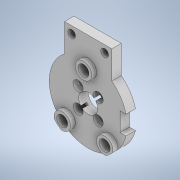
# Autodesk Inventor part: Spacerplate
Saved by Autodesk Inventor 2021 (Build 250183000, 183)
## iProperties
Created: 2024-03-24
Part Number: Spacerplate
Material: Generic
Document SubType Name: Modeling
Designer: Lukas
Density: 1 g/cm^3
Appearance: Default
Author: Lukas
Autodesk Inventor part; units mm, degrees
ref_plane "YZ Plane" through (0, 0, 0) normal (1, 0, 0) x (0, 1, 0)
ref_plane "XZ Plane" through (0, 0, 0) normal (0, 1, 0) x (-1, 0, 0)
ref_plane "XY Plane" through (0, 0, 0) normal (0, 0, 1) x (1, 0, 0)
sketch "Sketch1" plane through (0, 0, 0) normal (0, 0, 1) x (1, 0, 0)
  circle A0 centre (0, 0) radius 16.5
  circle A1 centre (-4.25, 4.25) radius 1.2
  circle A2 centre (-4.25, -4.25) radius 1.2
  circle A3 centre (4.25, -4.25) radius 1.2
  circle A4 centre (4.25, 4.25) radius 1.2
  circle A5 centre (0, 0) radius 4
  circle A6 centre (0, 13) radius 2.3
  circle A7 centre (-9, -10) radius 2.3
  circle A8 centre (9, -10) radius 2.3
  line L0 (16.5, -4) -> (13.5, -4)
  line L1 (13.5, -4) -> (13.5, 4)
  line L2 (13.5, 4) -> (16.5, 4)
  line L3 (16.5, 4) -> (16.5, -4)
  line L4 (-10, 13.1244) -> (-10, 25)
  line L5 (-10, 25) -> (10, 25)
  line L6 (10, 25) -> (10, 13.1244)
  circle A9 centre (7, 22) radius 1.6
  circle A10 centre (-7, 22) radius 1.6
  point P0 (13.5, 0)
  point P1 (16.0078, 4)
  point P2 (16.0078, -4)
  point P3 (0, 25)
  dimension "d0" = 33
  dimension "d1" = 8.5
  dimension "d2" = 8.5
  dimension "d3" = 4.25
  dimension "d4" = 4.25
  dimension "d5" = 2.4
  dimension "d6" = 8
  dimension "d7" = 13
  dimension "d8" = 4.6
  dimension "d9" = 10
  dimension "d10" = 9
  dimension "d11" = 9
  dimension "d17" = 3
  dimension "d18" = 8
  dimension "d27" = 25
  dimension "d28" = 20
  dimension "d30" = 3.2
  dimension "d31" = 14
  dimension "d32" = 7
  dimension "d33" = 3
  constraints: 14 end point, 11 centre point, 6 equal radius, 6 horizontal alignment, 4 vertical alignment, 2 coincident, 2 midpoint, 2 parallel, 2 perpendicular, 2 point on circle, 2 vertical, 1 horizontal, 1 tangent
  measures "d0" diameter of A0
  measures "d1" distance of A3.centre A4.centre
  measures "d2" distance of A1.centre A4.centre
  measures "d3" horizontal distance of A4.centre point (0, 0)
  measures "d4" horizontal distance of point (0, 0) A4.centre
  measures "d5" diameter of A4
  measures "d6" diameter of A5
  measures "d7" distance of A6.centre point (0, 0)
  measures "d8" diameter of A6
  measures "d9" vertical distance of point (0, 0) A7.centre
  measures "d10" horizontal distance of point (0, 0) A7.centre
  measures "d11" horizontal distance of point (0, 0) A8.centre
  measures "d17" distance of L0.start L0.end
  measures "d18" distance of L2.end L0.start
  measures "d27" distance from line of point (0, 0) L5
  measures "d28" distance of L4.end L5.end
  measures "d30" diameter of A9
  measures "d31" distance of A10.centre A9.centre
  measures "d32" horizontal distance of point (0, 0) A9.centre
  measures "d33" distance from line of L5 A9.centre
extrude "Extrusion1" add sketch "Sketch1" along normal blind 4 contours A0 L2 L1 L0 | A0 L4 L5 L6 picked at (-0.5777, -8.9613)
sketch "Sketch2" plane through (0, 0, 4) normal (0, 0, 1) x (0, -1, 0)
  circle A0 centre (-13, 0) radius 2.3 projected
  circle A1 centre (10, -9) radius 2.3 projected
  circle A2 centre (10, 9) radius 2.3 projected
  arc A3 (-13.1244, -10) -> (4, 16.0078) centre (0, 0) ccw projected
  circle A4 centre (-13, 0) radius 3.5
  circle A5 centre (10, 9) radius 3.5
  circle A6 centre (10, -9) radius 3.5
  point P0 (13.4568, -9.548)
  point P1 (10.9078, -12.3802)
  point P2 (10.9078, 12.3802)
  point P3 (13.4568, 9.548)
  dimension "d29" = 7
  constraints: 3 centre point, 3 coincident, 2 equal radius
  measures "d29" diameter of A4
extrude "Extrusion2" add sketch "Sketch2" along normal blind 2 contours A6 A3 | A5 A3 | A4 picked at (12.7903, -9.885) picked at (12.7903, 9.885)
sketch "Sketch3" plane through (0, 0, 4) normal (0, 0, 1) x (1, 0, 0)
  circle A0 centre (-4.25, 4.25) radius 1.2 projected
  circle A1 centre (-4.25, -4.25) radius 1.2 projected
  circle A2 centre (4.25, -4.25) radius 1.2 projected
  circle A3 centre (4.25, 4.25) radius 1.2 projected
  circle A4 centre (-4.25, 4.25) radius 2.1
  circle A5 centre (4.25, 4.25) radius 2.1
  circle A6 centre (4.25, -4.25) radius 2.1
  circle A7 centre (-4.25, -4.25) radius 2.1
  point P0 (0, 0)
  dimension "d19" = 4.2
  constraints: 4 centre point, 4 coincident, 3 equal radius
  measures "d19" diameter of A4
extrude "Extrusion3" cut sketch "Sketch3" against normal blind 2.5
ref_plane "Work Plane1" through (13.5, 4, 0) normal (0.9848078, 0.1736482, 0) x (0, 0, 1)
equation "\"d2\" = d1"
equation "\"d3\" = 0.5 * d1"
equation "\"d4\" = 0.5 * d2"
equation "\"d11\" = d10"
equation "\"d32\" = 0.5 * d31"
body "Solid1"
